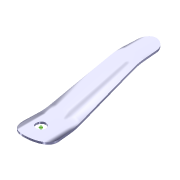
# Autodesk Inventor part: DS51F1496-08
Saved by Autodesk Inventor 2011 (Build 150239000, 239)
## iProperties
Manager: MANNY MANAGER
Company: ACME
Category: DATASETS
Created: 2009-12-09
Part Number: DS51F1496-08
Document SubType Name: Modeling
Designer: JOE DESIGNER
Density: 7.85 g/cm^3
Description: BACK SPRING
Stock Number: F1496
Project: IV2010 TO 2011 UPDATE
Checked By: CHUCK CHECKER
Engr Approved By: ED ENGINEER
Material: Steel
Mfg Approved By: DUNN RITE
Engineer: ERNIE ENGINEER
Mass: 3.52818 g
Surface Area: 12.738 cm^2
Volume: 0.449449 cm^3
Author: Joe Designer
Title: STILLSON WRENCH
Subject: Simplification for Simulation
Revision Number: 0
Comments: To use for Exercise: Rules Using Spreadsheets, Forms, and Triggers
Autodesk Inventor part; units mm, degrees
ref_plane "YZ Plane" through (0, 0, 0) normal (1, 0, 0) x (0, 1, 0)
ref_plane "XY Plane" through (0, 0, 0) normal (0, 0, 1) x (1, 0, 0)
sketch "Sketch1" plane through (0, 0, 0) normal (0, 0, 1) x (1, 0, 0)
  arc A0 (7.0946, 12.0692) -> (-7.0946, 12.0692) centre (0, 0) ccw
  arc A1 (7.5, 12.7589) -> (-7.5, 12.7589) centre (0, 0) ccw
  line L0 (7.0946, 12.0692) -> (7.5, 12.7589)
  line L1 (-7.5, 12.7589) -> (-7.0946, 12.0692)
  line L2 (-7.5, 14.8) -> (7.5, 14.8)
  point P0 (0, 14.8)
  dimension "d0" = 14
  dimension "d1" = 7.5
  dimension "d2" = 0.8
  dimension "d3" = 0.8
  constraints: 6 end point, 5 point on circle, 2 centre point, 2 vertical alignment, 1 coincident, 1 equal length, 1 horizontal, 1 midpoint, 1 tangent
  measures "d0" radius of A0
  measures "d1" distance of point (0, 14.8) L2.start
  measures "d2" distance of L1.start L1.end
  measures "d3" radial gap between concentric circles of A1 A0
sketch "Sketch2" plane through (0, 0, 0) normal (1, 0, 0) x (0, 0, -1)
  line L0 (0, 14) -> (0, 12.0692) construction
  line L1 (0, 12.0692) -> (12.5, 12.0692)
  line L2 (0, 12.0692) -> (12.5, 12.0692) construction
  arc A0 (12.5, 12.0692) -> (17.4305, 12.7184) centre (12.5, 31.1192) ccw
  line L3 (17.4305, 12.7184) -> (40.5695, 18.9184)
  arc A1 (45.5, 19.5675) -> (40.5695, 18.9184) centre (45.5, 0.5175) ccw
  line L4 (45.5, 19.5675) -> (55, 19.5675)
  point P0 (0, 0)
  dimension "d4" = 12.5
  dimension "d5" = 180
  dimension "d6" = 9.5
  dimension "d7" = 19.05
  dimension "d8" = 55
  dimension "d9" = 15
  constraints: 8 end point, 4 point on circle, 4 tangent, 2 centre point, 1 collinear, 1 equal radius, 1 horizontal, 1 parallel, 1 perpendicular
  measures "d4" distance of L0.end L1.end
  measures "d5" angle of L1 L2
  measures "d6" distance of L4.start L4.end
  measures "d7" radius of A0
  measures "d8" horizontal distance of L4.end L0.end
  measures "d9" angle of L3 L1
sweep "Sweep1" add profiles "Sketch1" path "Sketch2" keep normal constant yes
ref_plane "Work Plane1" through (0, 22.2983, -45.5) normal (0, 1, 0) x (-1, 0, 0)
sketch "Sketch3" plane through (0, 22.2983, -45.5) normal (0, 1, 0) x (0, 0, 1)
  line L0 (-5.7727, 3.9907) -> (38.0227, 6.9837)
  arc A0 (38.0227, -6.9837) -> (38.0227, 6.9837) centre (38.5, 0) ccw
  line L1 (38.0227, -6.9837) -> (-5.7727, -3.9907)
  arc A1 (-5.7727, 3.9907) -> (-5.7727, -3.9907) centre (-5.5, 0) ccw
  line L2 (-9.5, -7.5) -> (-9.5, 7.5) projected
  line L3 (45.5, -7.5) -> (45.5, 7.5) projected
  circle A2 centre (38.5, 0) radius 2
  point P0 (45.5, 0)
  point P1 (45.5, 0)
  point P2 (-9.5, 0)
  dimension "d11" = 4
  dimension "d12" = 7
  dimension "d14" = 4
  constraints: 6 tangent, 5 end point, 4 point on circle, 3 centre point, 2 horizontal alignment, 2 midpoint, 1 coincident
  measures "d11" radius of A1
  measures "d12" radius of A0
  measures "d14" diameter of A2
extrude "Extrusion1" cut sketch "Sketch3" against normal through all keep common part
equation "\"d3\" = d2"
body "Solid1"
